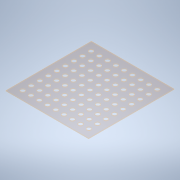
# Autodesk Inventor part: Electronics Base Plate
Saved by Autodesk Inventor 2022 (Build 260153000, 153)
## iProperties
Created: 2022-01-14
Part Number: Electronics Base Plate
Material: Generic
Document SubType Name: Modeling
Designer: merky
Density: 1 g/cm^3
Appearance: Polycarbonate - Smoked
Author: merky
Autodesk Inventor part; units mm, degrees
ref_plane "YZ Plane" through (0, 0, 0) normal (1, 0, 0) x (0, 1, 0)
ref_plane "XZ Plane" through (0, 0, 0) normal (0, 1, 0) x (-1, 0, 0)
ref_plane "XY Plane" through (0, 0, 0) normal (0, 0, 1) x (1, 0, 0)
sketch "Sketch4" plane through (0, 0, 0) normal (0, 1, 0) x (-1, 0, 0)
  circle A0 centre (38.1, -39.37) radius 9.525
  line L0 (0, 0) -> (0, -393.7)
  line L1 (381, 0) -> (0, 0)
  circle A1 centre (76.2, -39.37) radius 9.525
  circle A2 centre (114.3, -39.37) radius 9.525
  circle A3 centre (152.4, -39.37) radius 9.525
  circle A4 centre (190.5, -39.37) radius 9.525
  circle A5 centre (228.6, -39.37) radius 9.525
  circle A6 centre (266.7, -39.37) radius 9.525
  circle A7 centre (304.8, -39.37) radius 9.525
  circle A8 centre (342.9, -39.37) radius 9.525
  circle A9 centre (38.1, -78.74) radius 9.525
  circle A10 centre (76.2, -78.74) radius 9.525
  circle A11 centre (114.3, -78.74) radius 9.525
  circle A12 centre (152.4, -78.74) radius 9.525
  circle A13 centre (190.5, -78.74) radius 9.525
  circle A14 centre (228.6, -78.74) radius 9.525
  circle A15 centre (266.7, -78.74) radius 9.525
  circle A16 centre (304.8, -78.74) radius 9.525
  circle A17 centre (342.9, -78.74) radius 9.525
  circle A18 centre (38.1, -118.11) radius 9.525
  circle A19 centre (76.2, -118.11) radius 9.525
  circle A20 centre (114.3, -118.11) radius 9.525
  circle A21 centre (152.4, -118.11) radius 9.525
  circle A22 centre (190.5, -118.11) radius 9.525
  circle A23 centre (228.6, -118.11) radius 9.525
  circle A24 centre (266.7, -118.11) radius 9.525
  circle A25 centre (304.8, -118.11) radius 9.525
  circle A26 centre (342.9, -118.11) radius 9.525
  circle A27 centre (38.1, -157.48) radius 9.525
  circle A28 centre (76.2, -157.48) radius 9.525
  circle A29 centre (114.3, -157.48) radius 9.525
  circle A30 centre (152.4, -157.48) radius 9.525
  circle A31 centre (190.5, -157.48) radius 9.525
  circle A32 centre (228.6, -157.48) radius 9.525
  circle A33 centre (266.7, -157.48) radius 9.525
  circle A34 centre (304.8, -157.48) radius 9.525
  circle A35 centre (342.9, -157.48) radius 9.525
  circle A36 centre (38.1, -196.85) radius 9.525
  circle A37 centre (76.2, -196.85) radius 9.525
  circle A38 centre (114.3, -196.85) radius 9.525
  circle A39 centre (152.4, -196.85) radius 9.525
  circle A40 centre (190.5, -196.85) radius 9.525
  circle A41 centre (228.6, -196.85) radius 9.525
  circle A42 centre (266.7, -196.85) radius 9.525
  circle A43 centre (304.8, -196.85) radius 9.525
  circle A44 centre (342.9, -196.85) radius 9.525
  circle A45 centre (38.1, -236.22) radius 9.525
  circle A46 centre (76.2, -236.22) radius 9.525
  circle A47 centre (114.3, -236.22) radius 9.525
  circle A48 centre (152.4, -236.22) radius 9.525
  circle A49 centre (190.5, -236.22) radius 9.525
  circle A50 centre (228.6, -236.22) radius 9.525
  circle A51 centre (266.7, -236.22) radius 9.525
  circle A52 centre (304.8, -236.22) radius 9.525
  circle A53 centre (342.9, -236.22) radius 9.525
  circle A54 centre (38.1, -275.59) radius 9.525
  circle A55 centre (76.2, -275.59) radius 9.525
  circle A56 centre (114.3, -275.59) radius 9.525
  circle A57 centre (152.4, -275.59) radius 9.525
  circle A58 centre (190.5, -275.59) radius 9.525
  circle A59 centre (228.6, -275.59) radius 9.525
  circle A60 centre (266.7, -275.59) radius 9.525
  circle A61 centre (304.8, -275.59) radius 9.525
  circle A62 centre (342.9, -275.59) radius 9.525
  circle A63 centre (38.1, -314.96) radius 9.525
  circle A64 centre (76.2, -314.96) radius 9.525
  circle A65 centre (114.3, -314.96) radius 9.525
  circle A66 centre (152.4, -314.96) radius 9.525
  circle A67 centre (190.5, -314.96) radius 9.525
  circle A68 centre (228.6, -314.96) radius 9.525
  circle A69 centre (266.7, -314.96) radius 9.525
  circle A70 centre (304.8, -314.96) radius 9.525
  circle A71 centre (342.9, -314.96) radius 9.525
  circle A72 centre (38.1, -354.33) radius 9.525
  circle A73 centre (76.2, -354.33) radius 9.525
  circle A74 centre (114.3, -354.33) radius 9.525
  circle A75 centre (152.4, -354.33) radius 9.525
  circle A76 centre (190.5, -354.33) radius 9.525
  circle A77 centre (228.6, -354.33) radius 9.525
  circle A78 centre (266.7, -354.33) radius 9.525
  circle A79 centre (304.8, -354.33) radius 9.525
  circle A80 centre (342.9, -354.33) radius 9.525
  line L2 (0, 0) -> (381, 0)
  line L3 (381, 0) -> (381, -393.7)
  line L4 (381, -393.7) -> (0, -393.7)
  line L5 (0, -393.7) -> (0, 0)
  dimension "d52" = 19.05
  dimension "d53" = 38.1
  dimension "d54" = 39.37
  dimension "d55" = 38.1
  dimension "d56" = 39.37
  dimension "d57" = 381
  dimension "d58" = 393.7
  dimension "d59" = 39.37
  dimension "d60" = 38.1
  constraints: 81 centre point, 12 end point, 2 parallel, 1 horizontal, 1 perpendicular, 1 vertical, 160 other
  measures "d52" diameter of A0
  measures "d53" distance from line of L0 A0.centre
  measures "d54" distance from line of L1 A0.centre
  measures "d55" distance of A0.centre A1.centre
  measures "d56" distance of A0.centre A9.centre
  measures "d57" distance of L4.start L5.start
  measures "d58" distance of L2.end L4.start
  measures "d59" distance from line of L4 A80.centre
  measures "d60" distance from line of L3 A80.centre
extrude "Extrusion3" add sketch "Sketch4" along normal blind 3.175
body "Solid2"
